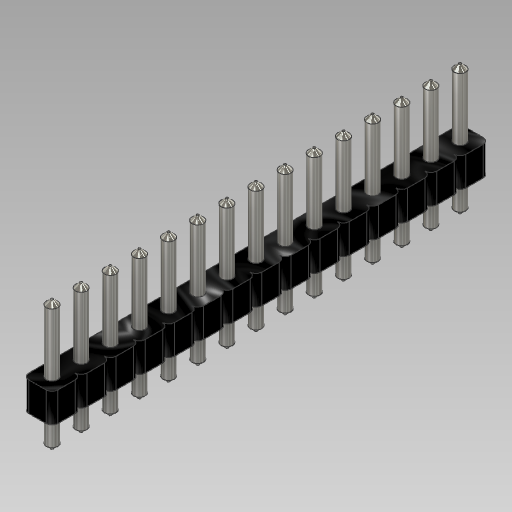
# Autodesk Inventor part: 15 pin header - round
Saved by Autodesk Inventor 2020 (Build 240168000, 168)
## iProperties
Created: 2017-10-26
Part Number: 15 pin header - round
Material: Generic
Document SubType Name: Modeling
Designer: Alex
Density: 1 g/cm^3
Appearance: Default
Author: Alex
Autodesk Inventor part; units mm, degrees
ref_plane "YZ Plane" through (0, 0, 0) normal (1, 0, 0) x (0, 1, 0)
ref_plane "XZ Plane" through (0, 0, 0) normal (0, 1, 0) x (-1, 0, 0)
ref_plane "XY Plane" through (0, 0, 0) normal (0, 0, 1) x (1, 0, 0)
sketch "Sketch1" plane through (0, 0, 0) normal (0, 1, 0) x (-1, 0, 0)
  line L0 (-0.762, -19.05) -> (0.762, -19.05)
  arc A0 (0.762, -19.05) -> (1.27, -18.542) centre (0.762, -18.542) ccw
  line L1 (1.27, -18.542) -> (1.27, -17.018)
  arc A1 (1.27, -17.018) -> (0.762, -16.51) centre (0.762, -17.018) ccw
  arc A2 (0.762, -16.51) -> (1.27, -16.002) centre (0.762, -16.002) ccw
  line L2 (1.27, -16.002) -> (1.27, -14.478)
  arc A3 (1.27, -14.478) -> (0.762, -13.97) centre (0.762, -14.478) ccw
  arc A4 (0.762, -13.97) -> (1.27, -13.462) centre (0.762, -13.462) ccw
  line L3 (1.27, -13.462) -> (1.27, -11.938)
  arc A5 (1.27, -11.938) -> (0.762, -11.43) centre (0.762, -11.938) ccw
  arc A6 (0.762, -11.43) -> (1.27, -10.922) centre (0.762, -10.922) ccw
  line L4 (1.27, -10.922) -> (1.27, -9.398)
  arc A7 (1.27, -9.398) -> (0.762, -8.89) centre (0.762, -9.398) ccw
  arc A8 (0.762, -8.89) -> (1.27, -8.382) centre (0.762, -8.382) ccw
  line L5 (1.27, -8.382) -> (1.27, -6.858)
  arc A9 (1.27, -6.858) -> (0.762, -6.35) centre (0.762, -6.858) ccw
  arc A10 (0.762, -6.35) -> (1.27, -5.842) centre (0.762, -5.842) ccw
  line L6 (1.27, -5.842) -> (1.27, -4.318)
  arc A11 (1.27, -4.318) -> (0.762, -3.81) centre (0.762, -4.318) ccw
  arc A12 (0.762, -3.81) -> (1.27, -3.302) centre (0.762, -3.302) ccw
  line L7 (1.27, -3.302) -> (1.27, -1.778)
  arc A13 (1.27, -1.778) -> (0.762, -1.27) centre (0.762, -1.778) ccw
  arc A14 (0.762, -1.27) -> (1.27, -0.762) centre (0.762, -0.762) ccw
  line L8 (1.27, -0.762) -> (1.27, 0.762)
  arc A15 (1.27, 0.762) -> (0.762, 1.27) centre (0.762, 0.762) ccw
  arc A16 (0.762, 1.27) -> (1.27, 1.778) centre (0.762, 1.778) ccw
  line L9 (1.27, 1.778) -> (1.27, 3.302)
  arc A17 (1.27, 3.302) -> (0.762, 3.81) centre (0.762, 3.302) ccw
  arc A18 (0.762, 3.81) -> (1.27, 4.318) centre (0.762, 4.318) ccw
  line L10 (1.27, 4.318) -> (1.27, 5.842)
  arc A19 (1.27, 5.842) -> (0.762, 6.35) centre (0.762, 5.842) ccw
  arc A20 (0.762, 6.35) -> (1.27, 6.858) centre (0.762, 6.858) ccw
  line L11 (1.27, 6.858) -> (1.27, 8.382)
  arc A21 (1.27, 8.382) -> (0.762, 8.89) centre (0.762, 8.382) ccw
  arc A22 (0.762, 8.89) -> (1.27, 9.398) centre (0.762, 9.398) ccw
  line L12 (1.27, 9.398) -> (1.27, 10.922)
  arc A23 (1.27, 10.922) -> (0.762, 11.43) centre (0.762, 10.922) ccw
  arc A24 (0.762, 11.43) -> (1.27, 11.938) centre (0.762, 11.938) ccw
  line L13 (1.27, 11.938) -> (1.27, 13.462)
  arc A25 (1.27, 13.462) -> (0.762, 13.97) centre (0.762, 13.462) ccw
  arc A26 (0.762, 13.97) -> (1.27, 14.478) centre (0.762, 14.478) ccw
  line L14 (1.27, 14.478) -> (1.27, 16.002)
  arc A27 (1.27, 16.002) -> (0.762, 16.51) centre (0.762, 16.002) ccw
  arc A28 (0.762, 16.51) -> (1.27, 17.018) centre (0.762, 17.018) ccw
  line L15 (1.27, 17.018) -> (1.27, 18.542)
  arc A29 (1.27, 18.542) -> (0.762, 19.05) centre (0.762, 18.542) ccw
  line L16 (0.762, 19.05) -> (-0.762, 19.05)
  arc A30 (-0.762, 19.05) -> (-1.27, 18.542) centre (-0.762, 18.542) ccw
  line L17 (-1.27, 18.542) -> (-1.27, 17.018)
  arc A31 (-1.27, 17.018) -> (-0.762, 16.51) centre (-0.762, 17.018) ccw
  arc A32 (-0.762, 16.51) -> (-1.27, 16.002) centre (-0.762, 16.002) ccw
  line L18 (-1.27, 16.002) -> (-1.27, 14.478)
  arc A33 (-1.27, 14.478) -> (-0.762, 13.97) centre (-0.762, 14.478) ccw
  arc A34 (-0.762, 13.97) -> (-1.27, 13.462) centre (-0.762, 13.462) ccw
  line L19 (-1.27, 13.462) -> (-1.27, 11.938)
  arc A35 (-1.27, 11.938) -> (-0.762, 11.43) centre (-0.762, 11.938) ccw
  arc A36 (-0.762, 11.43) -> (-1.27, 10.922) centre (-0.762, 10.922) ccw
  line L20 (-1.27, 10.922) -> (-1.27, 9.398)
  arc A37 (-1.27, 9.398) -> (-0.762, 8.89) centre (-0.762, 9.398) ccw
  arc A38 (-0.762, 8.89) -> (-1.27, 8.382) centre (-0.762, 8.382) ccw
  line L21 (-1.27, 8.382) -> (-1.27, 6.858)
  arc A39 (-1.27, 6.858) -> (-0.762, 6.35) centre (-0.762, 6.858) ccw
  arc A40 (-0.762, 6.35) -> (-1.27, 5.842) centre (-0.762, 5.842) ccw
  line L22 (-1.27, 5.842) -> (-1.27, 4.318)
  arc A41 (-1.27, 4.318) -> (-0.762, 3.81) centre (-0.762, 4.318) ccw
  arc A42 (-0.762, 3.81) -> (-1.27, 3.302) centre (-0.762, 3.302) ccw
  line L23 (-1.27, 3.302) -> (-1.27, 1.778)
  arc A43 (-1.27, 1.778) -> (-0.762, 1.27) centre (-0.762, 1.778) ccw
  arc A44 (-0.762, 1.27) -> (-1.27, 0.762) centre (-0.762, 0.762) ccw
  line L24 (-1.27, 0.762) -> (-1.27, -0.762)
  arc A45 (-1.27, -0.762) -> (-0.762, -1.27) centre (-0.762, -0.762) ccw
  arc A46 (-0.762, -1.27) -> (-1.27, -1.778) centre (-0.762, -1.778) ccw
  line L25 (-1.27, -1.778) -> (-1.27, -3.302)
  arc A47 (-1.27, -3.302) -> (-0.762, -3.81) centre (-0.762, -3.302) ccw
  arc A48 (-0.762, -3.81) -> (-1.27, -4.318) centre (-0.762, -4.318) ccw
  line L26 (-1.27, -4.318) -> (-1.27, -5.842)
  arc A49 (-1.27, -5.842) -> (-0.762, -6.35) centre (-0.762, -5.842) ccw
  arc A50 (-0.762, -6.35) -> (-1.27, -6.858) centre (-0.762, -6.858) ccw
  line L27 (-1.27, -6.858) -> (-1.27, -8.382)
  arc A51 (-1.27, -8.382) -> (-0.762, -8.89) centre (-0.762, -8.382) ccw
  arc A52 (-0.762, -8.89) -> (-1.27, -9.398) centre (-0.762, -9.398) ccw
  line L28 (-1.27, -9.398) -> (-1.27, -10.922)
  arc A53 (-1.27, -10.922) -> (-0.762, -11.43) centre (-0.762, -10.922) ccw
  arc A54 (-0.762, -11.43) -> (-1.27, -11.938) centre (-0.762, -11.938) ccw
  line L29 (-1.27, -11.938) -> (-1.27, -13.462)
  arc A55 (-1.27, -13.462) -> (-0.762, -13.97) centre (-0.762, -13.462) ccw
  arc A56 (-0.762, -13.97) -> (-1.27, -14.478) centre (-0.762, -14.478) ccw
  line L30 (-1.27, -14.478) -> (-1.27, -16.002)
  arc A57 (-1.27, -16.002) -> (-0.762, -16.51) centre (-0.762, -16.002) ccw
  arc A58 (-0.762, -16.51) -> (-1.27, -17.018) centre (-0.762, -17.018) ccw
  line L31 (-1.27, -17.018) -> (-1.27, -18.542)
  arc A59 (-1.27, -18.542) -> (-0.762, -19.05) centre (-0.762, -18.542) ccw
  line L32 (-1.27, 0) -> (1.27, 0) construction
  point P0 (0, 0)
  point P1 (0, -0.0199)
  point P2 (0, 0)
  constraints: 120 point on circle, 66 end point, 60 centre point, 3 midpoint
extrude "Extrusion1" add sketch "Sketch1" along normal mid plane 2.54
sketch "Sketch2" plane through (0, 1.27, 0) normal (0, 1, 0) x (1, 0, 0)
  circle A0 centre (0, 0) radius 0.508
  line L0 (-1.27, 0.762) -> (-1.27, -0.762) construction
  circle A1 centre (0, -2.54) radius 0.508
  circle A2 centre (0, -5.08) radius 0.508
  circle A3 centre (0, -7.62) radius 0.508
  circle A4 centre (0, -10.16) radius 0.508
  circle A5 centre (0, -12.7) radius 0.508
  circle A6 centre (0, -15.24) radius 0.508
  circle A7 centre (0, -17.78) radius 0.508
  circle A8 centre (0, 2.54) radius 0.508
  circle A9 centre (0, 0) radius 0.508
  circle A10 centre (0, -2.54) radius 0.508
  circle A11 centre (0, -5.08) radius 0.508
  circle A12 centre (0, -7.62) radius 0.508
  circle A13 centre (0, -10.16) radius 0.508
  circle A14 centre (0, -12.7) radius 0.508
  circle A15 centre (0, -15.24) radius 0.508
  circle A16 centre (0, 5.08) radius 0.508
  circle A17 centre (0, 2.54) radius 0.508
  circle A18 centre (0, 0) radius 0.508
  circle A19 centre (0, -2.54) radius 0.508
  circle A20 centre (0, -5.08) radius 0.508
  circle A21 centre (0, -7.62) radius 0.508
  circle A22 centre (0, -10.16) radius 0.508
  circle A23 centre (0, -12.7) radius 0.508
  circle A24 centre (0, 7.62) radius 0.508
  circle A25 centre (0, 5.08) radius 0.508
  circle A26 centre (0, 2.54) radius 0.508
  circle A27 centre (0, 0) radius 0.508
  circle A28 centre (0, -2.54) radius 0.508
  circle A29 centre (0, -5.08) radius 0.508
  circle A30 centre (0, -7.62) radius 0.508
  circle A31 centre (0, -10.16) radius 0.508
  circle A32 centre (0, 10.16) radius 0.508
  circle A33 centre (0, 7.62) radius 0.508
  circle A34 centre (0, 5.08) radius 0.508
  circle A35 centre (0, 2.54) radius 0.508
  circle A36 centre (0, 0) radius 0.508
  circle A37 centre (0, -2.54) radius 0.508
  circle A38 centre (0, -5.08) radius 0.508
  circle A39 centre (0, -7.62) radius 0.508
  circle A40 centre (0, 12.7) radius 0.508
  circle A41 centre (0, 10.16) radius 0.508
  circle A42 centre (0, 7.62) radius 0.508
  circle A43 centre (0, 5.08) radius 0.508
  circle A44 centre (0, 2.54) radius 0.508
  circle A45 centre (0, 0) radius 0.508
  circle A46 centre (0, -2.54) radius 0.508
  circle A47 centre (0, -5.08) radius 0.508
  circle A48 centre (0, 15.24) radius 0.508
  circle A49 centre (0, 12.7) radius 0.508
  circle A50 centre (0, 10.16) radius 0.508
  circle A51 centre (0, 7.62) radius 0.508
  circle A52 centre (0, 5.08) radius 0.508
  circle A53 centre (0, 2.54) radius 0.508
  circle A54 centre (0, 0) radius 0.508
  circle A55 centre (0, -2.54) radius 0.508
  circle A56 centre (0, 17.78) radius 0.508
  circle A57 centre (0, 15.24) radius 0.508
  circle A58 centre (0, 12.7) radius 0.508
  circle A59 centre (0, 10.16) radius 0.508
  circle A60 centre (0, 7.62) radius 0.508
  circle A61 centre (0, 5.08) radius 0.508
  circle A62 centre (0, 2.54) radius 0.508
  circle A63 centre (0, 0) radius 0.508
  dimension "d2" = 1.016
  dimension "d5" = 2.54
  dimension "d8" = 2.54
  constraints: 64 centre point, 2 vertical, 1 coincident, 126 other
  measures "d2" diameter of A0
  measures "d5" distance of A0.centre A1.centre
  measures "d8" distance of A0.centre A8.centre
extrude "Extrusion2" add sketch "Sketch2" along normal blind 5.842 and the other way blind 5.4356
chamfer "Chamfer1" distance 0.4064 angle 45 30 edges at (-0.508, 7.112, -7.62) (-0.508, 7.112, -2.54) (-0.508, 7.112, -10.16) (-0.508, 7.112, -5.08) (-0.508, 7.112, 10.16) (-0.508, 7.112, 5.08) (-0.508, 7.112, 0) (-0.508, 7.112, 2.54) (-0.508, 7.112, 7.62) (-0.508, 7.112, 15.24) (-0.508, 7.112, 12.7) (-0.508, 7.112, 17.78) (-0.508, 7.112, -17.78) (-0.508, 7.112, -12.7) (-0.508, 7.112, -15.24) (-0.508, -4.1656, -7.62) (-0.508, -4.1656, -2.54) (-0.508, -4.1656, -5.08) (-0.508, -4.1656, -10.16) (-0.508, -4.1656, 10.16) (-0.508, -4.1656, 5.08) (-0.508, -4.1656, 0) (-0.508, -4.1656, 2.54) (-0.508, -4.1656, 7.62) (-0.508, -4.1656, 15.24) (-0.508, -4.1656, 12.7) (-0.508, -4.1656, 17.78) (-0.508, -4.1656, -17.78) (-0.508, -4.1656, -12.7) (-0.508, -4.1656, -15.24)
body "Solid1"
